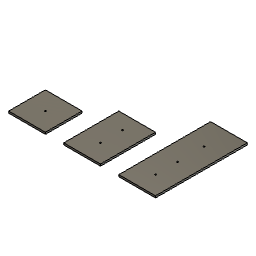
06-gear (Autodesk Fusion 360 design; units mm, degrees)
Autodesk Fusion 360 part; units mm, degrees
sketch "スケッチ1" plane through (0, 0, 0) normal (0, 1, 0) x (1, 0, 0)
  line L0 (0, 0) -> (50, 0)
  line L1 (50, 0) -> (50, 50)
  line L2 (50, 50) -> (0, 50)
  line L3 (0, 50) -> (0, 0)
  circle A0 centre (25, 25) radius 1
  line L4 (75, 0) -> (125, 0)
  line L5 (125, 0) -> (125, 75)
  line L6 (125, 75) -> (75, 75)
  line L7 (75, 75) -> (75, 0)
  line L8 (150, 0) -> (200, 0)
  line L9 (200, 0) -> (200, 125)
  line L10 (200, 125) -> (150, 125)
  line L11 (150, 125) -> (150, 0)
  circle A1 centre (100, 25) radius 1
  circle A2 centre (100, 55) radius 1
  circle A3 centre (175, 25) radius 1
  circle A4 centre (175, 55) radius 1
  circle A5 centre (175, 91) radius 1
  dimension "d1" = 2
  dimension "d4" = 2
  dimension "d5" = 2
  dimension "d6" = 2
  dimension "d7" = 2
  dimension "d8" = 2
  dimension "d9" = 36
  constraint horizontal L0
  constraint vertical L1
  constraint horizontal L2
  constraint vertical L3
  constraint coincident L0.start L3.end
  constraint horizontal L4
  constraint vertical L5
  constraint horizontal L6
  constraint vertical L7
  constraint horizontal L8
  constraint vertical L9
  constraint horizontal L10
  constraint vertical L11
  measures "d1" diameter of A0
  measures "d4" diameter of A1
  measures "d5" diameter of A2
  measures "d6" diameter of A3
  measures "d7" diameter of A4
  measures "d8" diameter of A5
  measures "d9" distance of A4.centre A5.centre
extrude "押し出し1" add sketch "スケッチ1" along normal blind 2.5 makes body 1 at (24.9751, 0, -41.9991) makes body 2 at (116.9787, 0, -33.4505) makes body 3 at (175, 0, -114)
